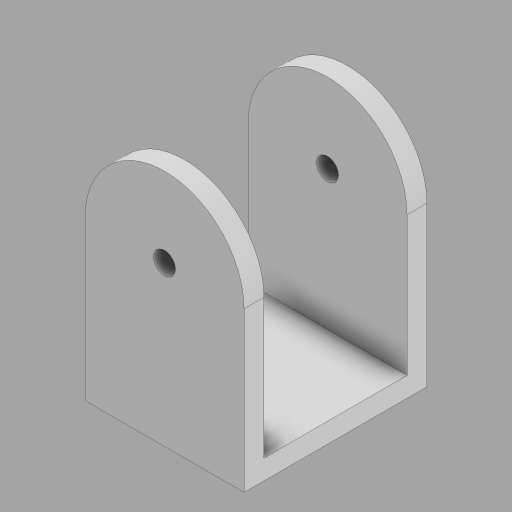
# Autodesk Inventor part: Apoio_Fixo_5040
Saved by Autodesk Inventor 2023.2 (Build 272271030, 271C)
## iProperties
Created: 2023-01-18
Part Number: Apoio_Fixo_5040
Material: Generic
Document SubType Name: Modeling
Designer: VICTOR
Density: 1 g/cm^3
Appearance: Default
Author: VICTOR
## iProperties of the stored document Apoio_Fixo_3DPrint.ipt
Created: 2023-05-17
Part Number: Apoio_Fixo_3DPrint
Material: Generic
Document SubType Name: Modeling
Designer: VICTOR
Density: 1 g/cm^3
Appearance: Default
Author: VICTOR
Autodesk Inventor part; units mm, degrees
ref_plane "YZ Plane" through (0, 0, 0) normal (1, 0, 0) x (0, 1, 0)
ref_plane "XZ Plane" through (0, 0, 0) normal (0, 1, 0) x (-1, 0, 0)
ref_plane "XY Plane" through (0, 0, 0) normal (0, 0, 1) x (1, 0, 0)
sketch "Sketch1" plane through (0, 0, 0) normal (0, 1, 0) x (-1, 0, 0)
  line L0 (0, 0) -> (40, 0)
  line L1 (40, 0) -> (40, -46)
  line L2 (40, -46) -> (0, -46)
  line L3 (0, -46) -> (0, 0)
  line L4 (40, 0) -> (0, 0)
  line L5 (0, 0) -> (0, -5)
  line L6 (0, -5) -> (40, -5)
  line L7 (40, -5) -> (40, 0)
  line L8 (40, -46) -> (0, -46)
  line L9 (0, -46) -> (0, -41)
  line L10 (0, -41) -> (40, -41)
  line L11 (40, -41) -> (40, -46)
  point P0 (40, -5)
  dimension "d1" = 40
  dimension "d2" = 46
  dimension "d3" = 5
  dimension "d4" = 5
  constraints: 24 end point, 6 parallel, 3 horizontal, 3 perpendicular, 2 point on line
  measures "d1" distance of L1.end L2.end
  measures "d2" distance of L0.end L1.end
  measures "d3" distance of L5.end L4.end
  measures "d4" distance of L8.end L9.end
extrude "Extrusion1" add sketch "Sketch1" along normal blind 5 contours L6 L1 L10 L3
extrude "Extrusion2" add sketch "Sketch1" along normal blind 60 contours L0 L1 L6 L3 | L10 L1 L2 L3
fillet "Fillet1" radius 20 4 edges at (-40, 60, -43.5) (0, 60, -43.5) (0, 60, -2.5) (-40, 60, -2.5)
sketch "Sketch2" plane through (0, 0, -46) normal (0, 0, -1) x (-1, 0, 0)
  arc A0 (40, 40) -> (0, 40) centre (20, 40) ccw projected
  line L0 (0, 0) -> (0, 40) projected
  line L1 (0, 0) -> (40, 0) projected
  line L2 (40, 0) -> (40, 40) projected
  circle A1 centre (20, 40) radius 2.75
  point P0 (0, 0)
  dimension "d10" = 5.5
  constraints: 1 centre point, 1 coincident
  measures "d10" diameter of A1
extrude "Extrusion3" cut sketch "Sketch2" against normal blind 600 contours A1
body "Solid1"
